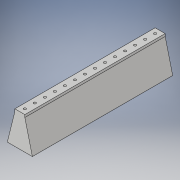
# Autodesk Inventor part: 22002102_Suppot Beam
Saved by Autodesk Inventor 2019.3 (Build 233278000, 278)
## iProperties
Created: 2019-01-16
Part Number: 22002102_Suppot Beam
Material: Všeobecné
Document SubType Name: Modeling
Designer: Ing. Martin Richter
Mass: 613251 g
Surface Area: 63633.2 cm^2
Volume: 613251 cm^3
Density: 1 g/cm^3
Appearance: Výchozí
Author: Ing. Martin Richter
Autodesk Inventor part; units mm, degrees
ref_plane "YZ Plane" through (0, 0, 0) normal (1, 0, 0) x (0, 1, 0)
ref_plane "XZ Plane" through (0, 0, 0) normal (0, 1, 0) x (-1, 0, 0)
ref_plane "XY Plane" through (0, 0, 0) normal (0, 0, 1) x (1, 0, 0)
sketch "Náčrt1" plane through (0, 0, 0) normal (0, 1, 0) x (1, 0, 0)
  line L0 (-250, 0) -> (250, 0)
  line L1 (250, 0) -> (100, -600)
  line L2 (100, -600) -> (100, -650)
  line L3 (100, -650) -> (-100, -650)
  line L4 (-100, -650) -> (-100, -600)
  line L5 (-100, -600) -> (-250, 0)
  point P0 (0, 0)
  point P1 (0, 0)
  point P2 (0, -650)
  dimension "d0" = 500
  dimension "d1" = 50
  dimension "d2" = 600
  dimension "d3" = 200
  constraints: 12 end point, 3 perpendicular, 2 midpoint, 1 coincident, 1 horizontal, 1 horizontal alignment, 1 vertical alignment
  measures "d0" distance of L0.start L0.end
  measures "d1" distance of L3.end L4.end
  measures "d2" vertical distance of L4.end L0.start
  measures "d3" distance of L2.end L3.end
extrude "Vysunutí1" add sketch "Náčrt1" along normal blind 2800
sketch "Náčrt2" plane through (-100, 0, 650) normal (0, 0, 1) x (1, 0, 0)
  line L0 (200, 0) -> (0, 0) construction
  line L1 (200, 0) -> (200, 2800) construction
  circle A0 centre (100, 100) radius 25
  circle A1 centre (100, 2700) radius 35.9949 construction
  line L2 (100, 100) -> (100, 2700) construction
  point P0 (100, 0)
  point P1 (100, 1400)
  point P2 (200, 1400)
  point P3 (100, 0)
  dimension "d6" = 2600
  dimension "d7" = 50
  constraints: 3 midpoint, 2 centre point, 2 end point, 1 horizontal alignment, 1 vertical, 1 vertical alignment
  measures "d6" distance of L2.start L2.end
  measures "d7" diameter of A0
extrude "Vysunutí2" cut sketch "Náčrt2" against normal blind 100
pattern_linear "Obdélníkové pole1" count 14 spacing 200 along (0, 1, 0) of "Vysunutí2"
